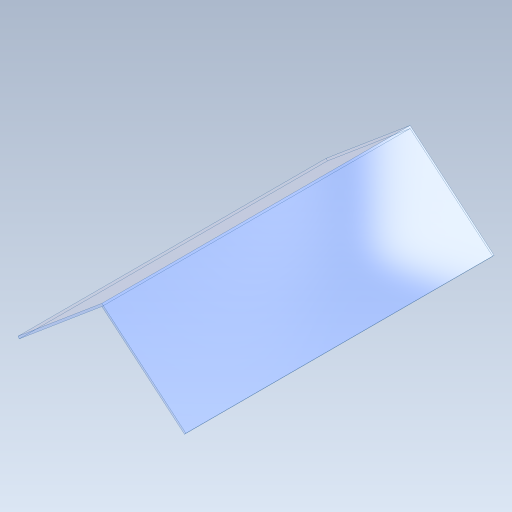
# Autodesk Inventor part: techo
Saved by Autodesk Inventor 2023 (Build 270158000, 158)
## iProperties
Created: 2023-03-17
Part Number: techo
Material: PET Plastic
Document SubType Name: Modeling
Designer: santi
Density: 1.541 g/cm^3
Appearance: Polycarbonate - Clear
Author: santi
Autodesk Inventor part; units mm, degrees
ref_plane "YZ Plane" through (0, 0, 0) normal (1, 0, 0) x (0, 1, 0)
ref_plane "XZ Plane" through (0, 0, 0) normal (0, 1, 0) x (-1, 0, 0)
ref_plane "XY Plane" through (0, 0, 0) normal (0, 0, 1) x (1, 0, 0)
sketch "Sketch1" plane through (0, 0, 0) normal (0, 0, 1) x (1, 0, 0)
  line L0 (0, 0) -> (80.4347, 67.4927)
  line L1 (80.4347, 67.4927) -> (160.8693, 0)
  line L2 (0, 0) -> (279.217, 0) construction
  line L3 (160.8693, 0) -> (162.1549, 1.5321)
  line L4 (162.1549, 1.5321) -> (80.4347, 70.1035)
  line L5 (-1.2856, 1.5321) -> (80.4347, 70.1035)
  line L6 (0, 0) -> (-1.2856, 1.5321)
  dimension "d0" = 105
  dimension "d1" = 105
  dimension "d2" = 100
  dimension "d3" = 2
  dimension "d4" = 90
  dimension "d7" = 2
  dimension "d8" = 90
  constraints: 14 end point, 2 parallel, 1 horizontal, 1 point on line
  measures "d0" distance of L0.start L0.end
  measures "d1" distance of L0.end L1.end
  measures "d2" angle of L1 L0
  measures "d3" distance of L1.end L3.end
  measures "d4" angle of L4 L3
  measures "d7" distance of L5.start L0.start
  measures "d8" angle of L6 L0
extrude "Extrusion1" add sketch "Sketch1" against normal blind 300
body "Solid1"
